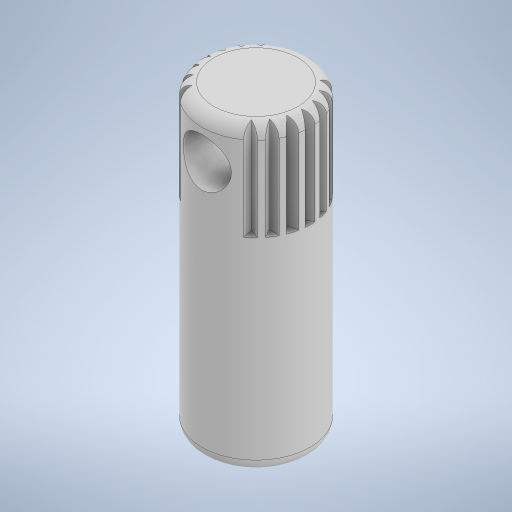
# Autodesk Inventor part: Llave 12MM
Saved by Autodesk Inventor 2024.2 (Build 282272000, 272)
## iProperties
Created: 2026-02-18
Part Number: Llave 12MM
Material: Generic
Document SubType Name: Modeling
Designer: ja.restrepo1
Density: 1 g/cm^3
Appearance: Default
Author: ja.restrepo1
Autodesk Inventor part; units mm, degrees
ref_plane "YZ Plane" through (0, 0, 0) normal (1, 0, 0) x (0, 1, 0)
ref_plane "XZ Plane" through (0, 0, 0) normal (0, 1, 0) x (-1, 0, 0)
ref_plane "XY Plane" through (0, 0, 0) normal (0, 0, 1) x (1, 0, 0)
sketch "Sketch1" plane through (0, 0, 0) normal (1, 0, 0) x (0, 1, 0)
  line L0 (25, 0) -> (-25, 0)
  line L1 (-25, 0) -> (-25, 7)
  line L2 (-23, 9) -> (0, 9)
  line L3 (0, 9) -> (23, 9)
  line L4 (25, 7) -> (25, 0)
  arc A0 (-23, 9) -> (-25, 7) centre (-23, 7) ccw
  arc A1 (25, 7) -> (23, 9) centre (23, 7) ccw
  point P0 (0, 0)
  point P1 (-25, 9)
  point P2 (25, 9)
  point P3 (0, 0)
  dimension "d0" = 50
  dimension "d1" = 9
  dimension "d2" = 25
  dimension "d3" = 180
  dimension "d8" = 2
  constraints: 10 end point, 4 point on circle, 4 point on line, 4 tangent, 2 centre point, 2 coincident, 2 perpendicular, 1 equal radius, 1 horizontal, 1 midpoint, 1 parallel
  measures "d0" distance of L0.start L0.end
  measures "d1" distance of L0.end point (-25, 9)
  measures "d2" distance of point (-25, 9) L2.end
  measures "d3" angle of L2 L3
  measures "d8" radius of A0
revolve "Revolution1" add sketch "Sketch1" angle 360 about axis through (0, 25, 0) along (0, -1, 0)
sketch "Sketch2" plane through (0, -25, 0) normal (0, -1, 0) x (1, 0, 0)
  line L0 (5.85, 3.3775) -> (5.85, -3.3775)
  line L1 (5.85, -3.3775) -> (0, -6.755)
  line L2 (0, -6.755) -> (-5.85, -3.3775)
  line L3 (-5.85, -3.3775) -> (-5.85, 3.3775)
  line L4 (-5.85, 3.3775) -> (0, 6.755)
  line L5 (0, 6.755) -> (5.85, 3.3775)
  circle A0 centre (0, 0) radius 2
  point P0 (0, 0)
  dimension "d5" = 11.7
  dimension "d13" = 4
  constraints: 12 end point, 2 coincident, 1 centre point, 1 vertical, 13 other
  measures "d5" distance between parallel lines of L3 L0
  measures "d13" diameter of A0
extrude "Extrusion1" cut sketch "Sketch2" against normal blind 7 contours L0 L1 L2 L3 L4 L5 | A0
sketch "Sketch3" plane through (0, 0, 0) normal (0, 0, 1) x (1, 0, 0)
  circle A0 centre (0, 18) radius 4
  point P0 (0, 0)
  dimension "d9" = 8
  dimension "d10" = 18
  constraints: 1 centre point, 1 vertical alignment
  measures "d9" diameter of A0
  measures "d10" distance of point (0, 0) A0.centre
extrude "Extrusion2" cut sketch "Sketch3" along normal through all both and the other way through all
extrude "Extrusion3" cut sketch "Sketch2" against normal blind 16 contours A0
chamfer "Chamfer1" distance 1.5 angle 75 1 edges at (-2, -18, 0) measured on face at (-2.5, -18, 0)
sketch "Sketch4" plane through (0, 25, 0) normal (0, 1, 0) x (1, 0, 0)
  line L0 (9.05, 0.866) -> (9.05, -0.866)
  line L1 (9.05, -0.866) -> (7.55, 0)
  line L2 (7.55, 0) -> (9.05, 0.866)
  line L3 (8.9274, 1.7187) -> (7.2442, 2.1271)
  line L4 (7.2442, 2.1271) -> (8.4394, 3.3806)
  line L5 (8.4394, 3.3806) -> (8.9274, 1.7187)
  line L6 (8.0816, 4.1643) -> (6.3515, 4.0818)
  line L7 (6.3515, 4.0818) -> (7.1451, 5.6213)
  line L8 (7.1451, 5.6213) -> (8.0816, 4.1643)
  line L9 (6.581, 6.2724) -> (4.9442, 5.7059)
  line L10 (4.9442, 5.7059) -> (5.272, 7.4067)
  line L11 (5.272, 7.4067) -> (6.581, 6.2724)
  line L12 (4.5473, 7.8724) -> (3.1364, 6.8677)
  line L13 (3.1364, 6.8677) -> (2.9717, 8.5919)
  line L14 (2.9717, 8.5919) -> (4.5473, 7.8724)
  line L15 (2.1452, 8.8346) -> (1.0745, 7.4732)
  line L16 (1.0745, 7.4732) -> (0.4307, 9.0811)
  line L17 (0.4307, 9.0811) -> (2.1452, 8.8346)
  line L18 (-0.4307, 9.0811) -> (-1.0745, 7.4732)
  line L19 (-1.0745, 7.4732) -> (-2.1452, 8.8346)
  line L20 (-2.1452, 8.8346) -> (-0.4307, 9.0811)
  line L21 (-2.9717, 8.5919) -> (-3.1364, 6.8677)
  line L22 (-3.1364, 6.8677) -> (-4.5473, 7.8724)
  line L23 (-4.5473, 7.8724) -> (-2.9717, 8.5919)
  line L24 (-5.272, 7.4067) -> (-4.9442, 5.7059)
  line L25 (-4.9442, 5.7059) -> (-6.581, 6.2724)
  line L26 (-6.581, 6.2724) -> (-5.272, 7.4067)
  line L27 (-7.1451, 5.6213) -> (-6.3515, 4.0818)
  line L28 (-6.3515, 4.0818) -> (-8.0816, 4.1643)
  line L29 (-8.0816, 4.1643) -> (-7.1451, 5.6213)
  line L30 (-8.4394, 3.3806) -> (-7.2442, 2.1271)
  line L31 (-7.2442, 2.1271) -> (-8.9274, 1.7187)
  line L32 (-8.9274, 1.7187) -> (-8.4394, 3.3806)
  line L33 (-9.05, 0.866) -> (-7.55, 0)
  line L34 (-7.55, 0) -> (-9.05, -0.866)
  line L35 (-9.05, -0.866) -> (-9.05, 0.866)
  line L36 (-8.9274, -1.7187) -> (-7.2442, -2.1271)
  line L37 (-7.2442, -2.1271) -> (-8.4394, -3.3806)
  line L38 (-8.4394, -3.3806) -> (-8.9274, -1.7187)
  line L39 (-8.0816, -4.1643) -> (-6.3515, -4.0818)
  line L40 (-6.3515, -4.0818) -> (-7.1451, -5.6213)
  line L41 (-7.1451, -5.6213) -> (-8.0816, -4.1643)
  line L42 (-6.581, -6.2724) -> (-4.9442, -5.7059)
  line L43 (-4.9442, -5.7059) -> (-5.272, -7.4067)
  line L44 (-5.272, -7.4067) -> (-6.581, -6.2724)
  line L45 (-4.5473, -7.8724) -> (-3.1364, -6.8677)
  line L46 (-3.1364, -6.8677) -> (-2.9717, -8.5919)
  line L47 (-2.9717, -8.5919) -> (-4.5473, -7.8724)
  line L48 (-2.1452, -8.8346) -> (-1.0745, -7.4732)
  line L49 (-1.0745, -7.4732) -> (-0.4307, -9.0811)
  line L50 (-0.4307, -9.0811) -> (-2.1452, -8.8346)
  line L51 (0.4307, -9.0811) -> (1.0745, -7.4732)
  line L52 (1.0745, -7.4732) -> (2.1452, -8.8346)
  line L53 (2.1452, -8.8346) -> (0.4307, -9.0811)
  line L54 (2.9717, -8.5919) -> (3.1364, -6.8677)
  line L55 (3.1364, -6.8677) -> (4.5473, -7.8724)
  line L56 (4.5473, -7.8724) -> (2.9717, -8.5919)
  line L57 (5.272, -7.4067) -> (4.9442, -5.7059)
  line L58 (4.9442, -5.7059) -> (6.581, -6.2724)
  line L59 (6.581, -6.2724) -> (5.272, -7.4067)
  line L60 (7.1451, -5.6213) -> (6.3515, -4.0818)
  line L61 (6.3515, -4.0818) -> (8.0816, -4.1643)
  line L62 (8.0816, -4.1643) -> (7.1451, -5.6213)
  line L63 (8.4394, -3.3806) -> (7.2442, -2.1271)
  line L64 (7.2442, -2.1271) -> (8.9274, -1.7187)
  line L65 (8.9274, -1.7187) -> (8.4394, -3.3806)
  point P0 (0, 0)
  point P1 (8.55, 0)
  dimension "d19" = 1.5
  dimension "d20" = 8.55
  dimension "d23" = 360
  constraints: 132 end point, 1 horizontal alignment, 1 vertical, 140 other
  measures "d19" distance from line of L1 L0.start
  measures "d20" distance of point (0, 0) point (8.55, 0)
extrude "Extrusion4" cut sketch "Sketch4" against normal blind 16 contours L0 L1 L2 | L3 L4 L5 | L6 L7 L8 | L9 L10 L11 | L24 L25 L26 | L27 L28 L29 | L30 L31 L32 | L33 L34 L35 | L36 L37 L38 | L39 L40 L41 | L42 L43 L44 | L57 L58 L59 | L60 L61 L62 | L63 L64 L65
body "Solid1"
